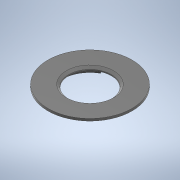
# Autodesk Inventor part: mirror_lock_v4
Saved by Autodesk Inventor 2020 (Build 240168000, 168)
## iProperties
Created: 2024-03-24
Part Number: mirror_lock_v4
Material: Типовые
Document SubType Name: Modeling
Designer: 4s
Density: 1 g/cm^3
Appearance: Гладкая — черная
Mass: 9.10734 g
Surface Area: 89.2393 cm^2
Volume: 9.10734 cm^3
Author: 4s
Autodesk Inventor part; units mm, degrees
ref_plane "YZ Plane" through (0, 0, 0) normal (1, 0, 0) x (0, 1, 0)
ref_plane "XZ Plane" through (0, 0, 0) normal (0, 1, 0) x (-1, 0, 0)
ref_plane "XY Plane" through (0, 0, 0) normal (0, 0, 1) x (1, 0, 0)
sketch "Эскиз1" plane through (0, 0, 0) normal (1, 0, 0) x (0, 1, 0)
  line L0 (0, 0) -> (10.522, 0) construction
  line L1 (0, 0) -> (0, -19) construction
  line L2 (0, 0) -> (0, -27.3) construction
  line L3 (0, -19) -> (3, -19)
  line L4 (3, -19) -> (3, -27.3)
  line L5 (3, -27.3) -> (0, -27.3)
  line L6 (0, -27.3) -> (0, -19)
  dimension "d0" = 19
  dimension "d1" = 27.3
  dimension "d2" = 3
  constraints: 14 end point, 2 horizontal, 2 parallel, 2 point on line, 1 perpendicular, 1 vertical
  measures "d0" distance of L0.start L1.end
  measures "d1" distance of L0.start L2.end
  measures "d2" distance of L4.end L5.end
revolve "Вращение1" add sketch "Эскиз1" angle 360 about axis through (0, 0, 0) along (0, 1, 0)
chamfer "Фаска1" distance 2 angle 45 1 edges at (0, 3, 19) measured on face at (0, 3, 19.5)
chamfer "Фаска2" distance 2 angle 45 1 edges at (0, 3, 27.3) measured on face at (0, 3, 26.8)
sketch "Эскиз2" plane through (0, 0, 0) normal (1, 0, 0) x (0, 1, 0)
  line L0 (0, 0) -> (7.8289, 0) construction
  line L1 (0, 0) -> (0, -24.8) construction
  line L2 (0, 27.3) -> (0, -27.3) construction
  line L3 (0, -25.2) -> (-3.7641, -25.2)
  line L4 (0, -27.3) -> (-3.7577, -27.3)
  line L5 (-4.0173, -25.2) -> (-4.0173, -26.7) construction
  line L6 (0, -25.2) -> (0, -27.3)
  line L7 (-6, 0.25) -> (-6, -25) construction
  line L8 (-6, -25) -> (-6, -25) construction
  arc A0 (-4.1761, -24.9833) -> (-5.6524, -26.3078) centre (-5, -25.55) ccw
  line L9 (-6, -25) -> (-6, 0) construction
  line L10 (-6, -24.55) -> (-6, -24.55) construction
  line L11 (-4.0173, -25.2) -> (-4.0633, -25.2) construction
  arc A1 (-4.0173, -25.7353) -> (-4.0633, -25.2) centre (-5, -25.55) ccw construction
  arc A2 (-4.1761, -24.9833) -> (-3.7641, -25.2) centre (-3.7641, -24.7) ccw
  line L12 (-5.0626, -26.8157) -> (-5.6524, -26.3078)
  arc A3 (-5.6524, -26.3078) -> (-4.0173, -25.7353) centre (-5, -25.55) ccw construction
  arc A4 (-5.0626, -26.8157) -> (-3.7577, -27.3) centre (-3.7577, -25.3) ccw
  point P0 (-4.1648, -25)
  point P1 (-4.5, -27.3)
  dimension "d10" = 24.8
  dimension "d11" = 4.0173
  dimension "d12" = 0.4
  dimension "d14" = 6
  dimension "d15" = 2
  dimension "d16" = 0
  dimension "d17" = 0.45
  dimension "d18" = 0.5
  dimension "d19" = 50
  dimension "d21" = 4.5
  dimension "d22" = 2
  dimension "d33" = 5
  constraints: 24 end point, 13 point on circle, 10 point on line, 10 tangent, 6 horizontal, 5 centre point, 3 vertical, 1 collinear, 1 midpoint
  measures "d10" distance of L0.start L1.end
  measures "d11" distance of L3.start L5.start
  measures "d12" distance from line of L1.end L3
  measures "d14" distance between parallel lines of L1 L7
  measures "d15" diameter of A0
  measures "d16" distance between parallel lines of L7 L9
  measures "d17" distance from line of point (-4.165, -25) L10
  measures "d18" radius of A2
  measures "d19" diameter of L8 L0
  measures "d21" distance of L2.end point (-4.5, -27.3)
  measures "d22" radius of A4
  measures "d33" distance from line of L6 A0.centre
revolve "Вращение2" add sketch "Эскиз2" angle 60 about axis through (0, 0, 0) along (0, -1, 0)
pattern_circular "Круговой массив1" count 4 over 360 about axis through (0, 1.5, 0) along (0, -1, 0) of "Вращение2"
sketch "Эскиз3" plane through (0, 3, 0) normal (0, 1, 0) x (1, 0, 0)
  circle A0 centre (0, 0) radius 21 construction
  circle A1 centre (0, 0) radius 25.3 projected
  circle A2 centre (0, 0) radius 19 construction
  circle A3 centre (0, 0) radius 21 construction
  arc A4 (-13.1539, 22.7833) -> (-26.3078, 0) centre (0, 0) ccw construction
  circle A5 centre (0, 0) radius 27.3 construction
  circle A6 centre (0, 0) radius 25.3 construction
  circle A7 centre (0, 0) radius 27.3 construction
  circle A8 centre (0, 0) radius 37.5
  dimension "d27" = 75
  constraints: 1 centre point, 1 coincident
  measures "d27" diameter of A8
extrude "Выдавливание1" add sketch "Эскиз3" against normal blind 2
sketch "Эскиз4" plane through (0, 0, -27.3) normal (0, -1, 0) x (1, 0, 0)
  circle A0 centre (0, 27.3) radius 25
  circle A1 centre (0, 27.3) radius 37.5 construction
  circle A2 centre (0, 27.3) radius 27.3 projected
  dimension "d30" = 50
  constraints: 1 centre point, 1 coincident
  measures "d30" diameter of A0
extrude "Выдавливание2" add sketch "Эскиз4" along normal blind 1.5
